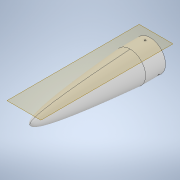
# Autodesk Inventor part: Spitze
Saved by Autodesk Inventor 2020 (Build 240168000, 168)
## iProperties
Created: 2022-01-25
Part Number: Spitze
Material: Generisch
Document SubType Name: Modeling
Designer: sp
Density: 1 g/cm^3
Appearance: Vorgabe
Author: sp
## iProperties of the stored document _3D-Druck.ipt
Created: 2022-05-21
Part Number: _3D-Druck
Material: Generisch
Document SubType Name: Modeling
Designer: sp
Density: 1 g/cm^3
Appearance: Vorgabe
Author: sp
Autodesk Inventor part; units mm, degrees
ref_plane "YZ Plane" through (0, 0, 0) normal (1, 0, 0) x (0, 1, 0)
ref_plane "XY Plane" through (0, 0, 0) normal (0, 0, 1) x (1, 0, 0)
sketch "Skizze1" plane through (0, 0, 0) normal (1, 0, 0) x (0, 1, 0)
  line L0 (0, 2094.1927) -> (0, -1699.1575) construction
  line L1 (933.6484, 0) -> (-899.755, 0) construction
  spline S0 degree 2 poles (29, 0) (0, 400) (-29, 0) knots 0 0 0 1 1 1
  line L2 (0, 90.8614) -> (0, 0)
  line L3 (0, 0) -> (44.134, 0)
  line L4 (30.9948, 0.1446) -> (30.9948, 0)
  line L5 (-30.9948, 0.1446) -> (-30.9948, 0)
  line L6 (0, 202) -> (0, 200)
  spline S1 degree 5 poles (30.9948, 0.1446) (30.6084, 5.4743) (30.2156, 10.8034) (29.8159, 16.1321) (29.0309, 26.4107) (28.2164, 36.6871) (27.8168, 41.6359) (27.0329, 51.1552) (26.2172, 60.6717) (25.8176, 65.2408) (25.035, 74.001) (24.2178, 82.758) (23.8183, 86.9475) (23.0372, 94.9478) (22.2185, 102.9442) (21.819, 106.7532) (21.04, 113.9939) (20.2193, 121.23) (19.8199, 124.6596) (19.043, 131.1427) (18.2197, 137.6201) (17.8203, 140.6709) (17.0461, 146.3979) (16.2194, 152.1176) (15.82, 154.7902) (15.049, 159.7622) (14.2179, 164.7245) (13.8185, 167.0191) (13.0516, 171.2394) (12.2141, 175.4462) (11.8142, 177.3653) (11.0516, 180.8421) (10.2037, 184.2991) (9.8023, 185.8469) (9.0423, 188.5964) (8.1747, 191.3135) (7.768, 192.4992) (6.9985, 194.5612) (6.0833, 196.5632) (5.6546, 197.4072) (4.7998, 198.8978) (3.715, 200.226) (3.1745, 200.7758) (1.9195, 201.7067) (0.4032, 202.0932) (-0.4032, 202.0932) (-1.9195, 201.7067) (-3.1745, 200.7758) (-3.715, 200.226) (-4.7998, 198.8978) (-5.6546, 197.4072) (-6.0833, 196.5632) (-6.9985, 194.5612) (-7.768, 192.4992) (-8.1747, 191.3135) (-9.0423, 188.5964) (-9.8023, 185.8469) (-10.2037, 184.2991) (-11.0516, 180.8421) (-11.8142, 177.3653) (-12.2141, 175.4462) (-13.0516, 171.2394) (-13.8185, 167.0191) (-14.2179, 164.7245) (-15.049, 159.7622) (-15.82, 154.7902) (-16.2194, 152.1176) (-17.0461, 146.3979) (-17.8203, 140.6709) (-18.2197, 137.6201) (-19.043, 131.1427) (-19.8199, 124.6596) (-20.2193, 121.23) (-21.04, 113.9939) (-21.819, 106.7532) (-22.2185, 102.9442) (-23.0372, 94.9478) (-23.8183, 86.9475) (-24.2178, 82.758) (-25.035, 74.001) (-25.8176, 65.2408) (-26.2172, 60.6717) (-27.0329, 51.1552) (-27.8168, 41.6359) (-28.2164, 36.6871) (-29.0309, 26.4107) (-29.8159, 16.1321) (-30.2156, 10.8034) (-30.6084, 5.4743) (-30.9948, 0.1446) knots 0 0 0 0 0 0 0.064534 0.064534 0.064534 0.124494 0.124494 0.124494 0.179885 0.179885 0.179885 0.23071 0.23071 0.23071 0.276961 0.276961 0.276961 0.318659 0.318659 0.318659 0.355817 0.355817 0.355817 0.388451 0.388451 0.388451 0.416579 0.416579 0.416579 0.440252 0.440252 0.440252 0.459561 0.459561 0.459561 0.474693 0.474693 0.474693 0.486125 0.486125 0.486125 0.495355 0.495355 0.495355 0.504645 0.504645 0.504645 0.513875 0.513875 0.513875 0.525307 0.525307 0.525307 0.540439 0.540439 0.540439 0.559748 0.559748 0.559748 0.583421 0.583421 0.583421 0.611549 0.611549 0.611549 0.644183 0.644183 0.644183 0.681341 0.681341 0.681341 0.723039 0.723039 0.723039 0.76929 0.76929 0.76929 0.820115 0.820115 0.820115 0.875506 0.875506 0.875506 0.935466 0.935466 0.935466 1 1 1 1 1 1
  point P0 (0, 82)
  point P1 (0, 80)
  point P2 (29, 0)
  dimension "d5" = 2
  dimension "d2" = 200
  dimension "d3" = 29
  dimension "d4" = 29
  constraints: 14 end point, 9 point on line, 3 perpendicular, 1 collinear, 1 horizontal, 1 vertical, 7 other
  measures "d2" distance of L6.end L2.end
  measures "d3" distance of L2.end point (29, 0)
  measures "d4" distance of point (-29, 0) L2.end
revolve "Umdrehung2" add sketch "Skizze1" angle 360 about axis through (0, 0, 90.8614) along (0, 0, -1)
sketch "Skizze2" plane through (0, 0, 0) normal (0, 0, -1) x (-1, 0, 0)
  circle A0 centre (0, 0) radius 29
  circle A1 centre (0, 0) radius 30.9948
  point P0 (0, 0)
  dimension "d17" = 58
  constraints: 2 centre point, 2 coincident
  measures "d17" diameter of A0
extrude "Extrusion1" add sketch "Skizze2" along normal blind 40
sketch "Skizze5" plane through (0, 0, -40) normal (0, 0, -1) x (-1, 0, 0)
  circle A0 centre (0, 0) radius 29
  circle A1 centre (0, 0) radius 30
  dimension "d19" = 60
  constraints: 2 centre point, 2 coincident
  measures "d19" diameter of A1
extrude "Extrusion3" cut sketch "Skizze5" against normal blind 5
ref_plane "Arbeitsebene3" through (0, 31, 0) normal (0, 1, 0) x (-1, 0, 0)
sketch "Skizze6" plane through (0, 31, 0) normal (0, 1, 0) x (-1, 0, 0)
  line L0 (0, -6.6699) -> (0, 5.8386) construction
  circle A0 centre (0, -30) radius 1.5
  line L1 (-30.9948, -40) -> (30.9948, -40) projected
  point P0 (0, 0)
  dimension "d23" = 3
  dimension "d24" = 10
  constraints: 2 end point, 2 point on line, 1 centre point, 1 vertical
  measures "d23" diameter of A0
  measures "d24" distance from line of L1 A0.centre
extrude "Extrusion4" cut sketch "Skizze6" against normal blind 5
pattern_circular "Runde Anordnung3" count 3 over 360 about axis through (0, 0, -10) along (0, 0, 1) of "Extrusion4"
